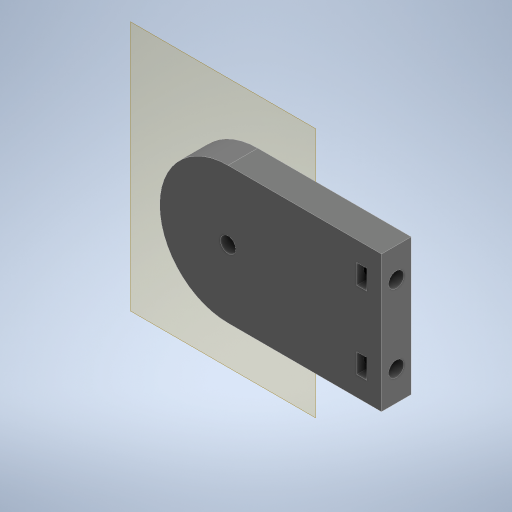
# Autodesk Inventor part: 6
Saved by Autodesk Inventor 2024.3 (Build 283343000, 343)
## iProperties
Created: 2024-09-05
Part Number: 6
Material: 아크릴, 선명
Document SubType Name: Modeling
Designer: 구지현
Density: 1.19 g/cm^3
Appearance: 회색
Mass: 7.93302 g
Surface Area: 33.8818 cm^2
Volume: 6.66641 cm^3
Author: 구지현
Autodesk Inventor part; units mm, degrees
ref_plane "YZ Plane" through (0, 0, 0) normal (1, 0, 0) x (0, 1, 0)
ref_plane "XZ Plane" through (0, 0, 0) normal (0, 1, 0) x (-1, 0, 0)
ref_plane "XY Plane" through (0, 0, 0) normal (0, 0, 1) x (1, 0, 0)
ref_plane "작업 평면1" through (0, 0, 0) normal (0, 0, 1) x (1, 0, 0)
sketch "스케치1" plane through (0, 0, 0) normal (0, 0, 1) x (1, 0, 0)
  line L0 (6.993261, -11.657355) -> (26.993258, -11.667122)
  arc A0 (7.006739, 15.942642) -> (6.993261, -11.657355) centre (7, 2.142643) ccw
  line L1 (27.006737, 15.932875) -> (7.006739, 15.942642)
  line L2 (26.993258, -11.667122) -> (27.006737, 15.932875)
  circle A1 centre (-0.776779, -5.636927) radius 1.65
  circle A2 centre (-4, 2.140669) radius 1.65
  circle A3 centre (-0.77957, 9.919422) radius 1.65
  circle A4 centre (6.998026, 13.142643) radius 1.65
  circle A5 centre (14.776779, 9.922214) radius 1.65
  circle A6 centre (18, 2.144617) radius 1.65
  circle A7 centre (14.77957, -5.634135) radius 1.65
  circle A8 centre (7.001974, -8.857357) radius 1.65
  circle A9 centre (7, 2.142643) radius 5.1
  circle A10 centre (7, 2.142643) radius 3.55
  line L3 (6.99331, -11.557355) -> (26.993307, -11.567122)
  line L4 (26.993307, -11.567122) -> (27.006786, 16.032875)
  line L5 (27.006786, 16.032875) -> (7.006788, 16.042642)
  arc A11 (7.006788, 16.042642) -> (6.99331, -11.557355) centre (7.000049, 2.242643) ccw
  circle A12 centre (-0.781923, -5.531732) radius 1.65
  circle A13 centre (-3.99995, 2.248015) radius 1.65
  circle A14 centre (-0.774326, 10.024615) radius 1.65
  circle A15 centre (7.005421, 13.242642) radius 1.65
  circle A16 centre (14.782021, 10.017018) radius 1.65
  circle A17 centre (18.000048, 2.237271) radius 1.65
  circle A18 centre (14.774424, -5.539329) radius 1.65
  circle A19 centre (6.994677, -8.757356) radius 1.65
  circle A20 centre (7.000049, 2.242643) radius 5.1
  point P0 (0, 0)
  dimension "d0" = 7.1
  constraints: 1 centre point, 1 coincident
  measures "d0" diameter of A10
extrude "돌출1" add sketch "스케치1" along normal blind 6 contours A11 L5 L4 L1 A0 | A0 L1 L2 L3 A11 | A1 A12 | A12 A1 | A1 A12 | A2 A13 | A13 A2 | A2 A13 | A14 A3 | A3 A14 | A3 A14 | A4 A15 | A4 A15 | A15 A4 | A5 A16 | A5 A16 | A16 A5 | A6 | A7 A18 | A18 A7 | A7 A18 | A8 A19 | A19 A8 | A8 A19 | A20 A9 | A9 A20 | A9 A20 | A17
offset faces "크기1" outward 2 faces at (10.504028, 1.573183, 4)
move faces "이동1" translate (4.999999, -0.002442, 0) faces at (27.00226, 6.766209, 4)
move faces "이동2" translate (1, -0.000488, 0) faces at (32.006753, 15.963766, 2) (32.00226, 6.763767, 4)
move faces "이동3" translate (4.999999, -0.002442, 0) faces at (33.006752, 15.963278, 2) (32.997783, -2.403387, 4)
sketch "스케치3" plane through (38.006784, 16.027503, 6) normal (0.9999999, -0.0004883, 0) x (0, 0, -1)
  circle A0 centre (3, -6) radius 1.55
  circle A1 centre (57.100995, -6.1) radius 1.55
  circle A2 centre (3, -21.6) radius 1.55
  circle A3 centre (57.100995, -21.7) radius 1.55
  line L0 (-17.781018, 8.082697) -> (114.718982, 8.082697)
  line L1 (-17.781018, -71.417303) -> (-17.781018, 8.082697)
  line L2 (114.718982, -71.417303) -> (-17.781018, -71.417303)
  line L3 (114.718982, 8.082697) -> (114.718982, -71.417303)
  point P0 (6, -16.046061)
extrude "돌출3" cut sketch "스케치3" against normal blind 10 contours A0 | A2
sketch "스케치4" plane through (0, 0, 0) normal (0, 0, -1) x (-1, 0, 0)
  line L0 (-38.006784, 16.027503) -> (-7.006788, 16.042642)
  line L1 (-33.358652, 16.029773) -> (-33.358652, 12.029773)
  line L2 (-33.358652, 16.029773) -> (-29.358652, 16.029773) construction
  line L3 (-6.99331, -11.557355) -> (-37.993306, -11.572494)
  line L4 (-34.023529, -11.570555) -> (-34.023529, -7.570555)
  line L5 (-34.023529, -11.570555) -> (-30.023529, -11.570555) construction
  line L6 (-37.993306, -11.572494) -> (-38.006784, 16.027503)
  line L7 (-37.995039, -8.023851) -> (-34.995039, -8.023851)
  line L8 (-37.995039, -8.023851) -> (-34.995039, -8.023851) construction
  line L9 (-34.995039, -7.570555) -> (-32.995039, -7.570555)
  line L10 (-32.995039, -7.570555) -> (-32.995039, -3.570555)
  line L11 (-32.995039, -3.570555) -> (-34.995039, -3.570555)
  line L12 (-34.995039, -3.570555) -> (-34.995039, -7.570555)
  line L13 (-34.995039, 12.029773) -> (-32.995039, 12.029773)
  line L14 (-32.995039, 12.029773) -> (-32.995039, 8.029773)
  line L15 (-32.995039, 8.029773) -> (-34.995039, 8.029773)
  line L16 (-34.995039, 8.029773) -> (-34.995039, 12.029773)
  point P0 (0, 0)
  dimension "d17" = 4
  dimension "d18" = 90
  dimension "d19" = 4
  dimension "d20" = 90
  dimension "d21" = 3
  dimension "d22" = 0
  dimension "d23" = 2
  dimension "d24" = 4
  dimension "d25" = 2
  dimension "d26" = 4
  constraints: 28 end point, 6 horizontal, 4 parallel, 4 point on line, 3 equal length, 2 perpendicular, 2 vertical
  measures "d17" distance of L1.start L1.end
  measures "d18" angle of L1 L2
  measures "d19" distance of L4.start L4.end
  measures "d20" angle of L5 L4
  measures "d21" distance of L7.start L7.end
  measures "d22" distance between parallel lines of L7 L8
  measures "d23" distance of L11.end L10.end
  measures "d24" distance of L10.end L9.end
  measures "d25" distance of L14.end L15.end
  measures "d26" distance of L13.end L14.end
extrude "돌출4" cut sketch "스케치4" against normal blind 10
